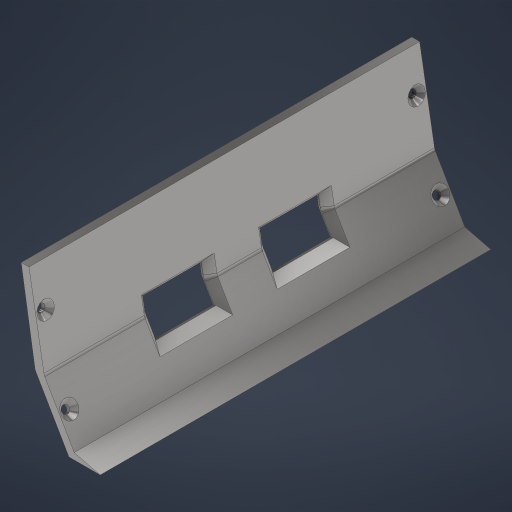
# Autodesk Inventor part: lemiesz
Saved by Autodesk Inventor 2024 (Build 280153000, 153)
## iProperties
Created: 2024-05-24
Part Number: lemiesz
Material: Steel
Document SubType Name: Modeling
Designer: Adam
Density: 7.85 g/cm^3
Appearance: Plate
Mass: 65.3515 g
Surface Area: 95.4294 cm^2
Volume: 8.32503 cm^3
Author: Adam
Autodesk Inventor part; units mm, degrees
ref_plane "YZ Plane" through (0, 0, 0) normal (1, 0, 0) x (0, 1, 0)
ref_plane "XZ Plane" through (0, 0, 0) normal (0, 1, 0) x (-1, 0, 0)
ref_plane "XY Plane" through (0, 0, 0) normal (0, 0, 1) x (1, 0, 0)
sketch "Sketch1" plane through (0, 0, 0) normal (0, 0, 1) x (1, 0, 0)
  line L0 (0, 0) -> (-8, 0)
  line L1 (-8, 0) -> (-16.4769, 14.6824)
  line L2 (0, 0) -> (-6.6505, 1.6626)
  line L3 (-14.1745, 14.6946) -> (-6.6505, 1.6626)
  line L4 (-14.4121, 15.3473) -> (-18.23, 37)
  line L5 (-14.3509, 15) -> (7.6359, 15) construction
  line L6 (-18.23, 37) -> (-20.23, 37)
  line L7 (-20.23, 37) -> (-16.719, 15.362)
  arc A0 (-16.719, 15.362) -> (-16.4769, 14.6824) centre (-14.7448, 15.6824) ccw
  arc A1 (-14.4121, 15.3473) -> (-14.1745, 14.6946) centre (-12.4425, 15.6946) ccw
  dimension "d0" = 8
  dimension "d1" = 120
  dimension "d3" = 2
  dimension "d37" = 100
  dimension "d38" = 2
  dimension "d39" = 2
  constraints: 16 end point, 4 point on circle, 4 tangent, 3 horizontal, 2 centre point, 2 point on line, 1 coincident, 1 equal length, 1 equal radius, 1 parallel
  measures "d0" distance of L0.start L1.start
  measures "d1" angle of L0 L1
  measures "d3" distance between parallel lines of L3 L1
  measures "d37" angle of L5 L4
  measures "d38" distance of L4.end L6.end
  measures "d39" radius of A0
extrude "Extrusion1" add sketch "Sketch1" along normal mid plane 100
sketch "Sketch6" plane through (0, 0, 0) normal (1, 0, 0) x (0, 1, 0)
  line L0 (1.6626, -50) -> (1.6626, 50) projected
  line L1 (17.6987, 22.5) -> (9.6987, 22.5)
  line L2 (9.6987, 22.5) -> (9.6987, 7.5)
  line L3 (9.6987, 7.5) -> (17.6987, 7.5)
  line L4 (17.6987, 7.5) -> (17.6987, 22.5)
  line L5 (17.6987, 22.5) -> (9.6987, 7.5) construction
  line L6 (9.6987, 22.5) -> (17.6987, 7.5) construction
  line L7 (17.6987, -7.5) -> (9.6987, -7.5)
  line L8 (9.6987, -7.5) -> (9.6987, -22.5)
  line L9 (9.6987, -22.5) -> (17.6987, -22.5)
  line L10 (17.6987, -22.5) -> (17.6987, -7.5)
  line L11 (17.6987, -7.5) -> (9.6987, -22.5) construction
  line L12 (9.6987, -7.5) -> (17.6987, -22.5) construction
  line L13 (1.6626, 50) -> (14.6946, 50) projected
  line L14 (14.6946, -50) -> (1.6626, -50) projected
  point P0 (0, 0)
  point P1 (37, 50)
  point P2 (34, 50)
  point P3 (13.6987, 15)
  point P4 (13.6987, -15)
  dimension "d22" = 8
  dimension "d23" = 15
  dimension "d24" = 8
  dimension "d25" = 15
  dimension "d40" = 35
  dimension "d41" = 35
  constraints: 24 end point, 4 midpoint, 4 parallel, 2 horizontal, 2 perpendicular
  measures "d22" distance of L3.end L2.end
  measures "d23" distance of L2.end L1.end
  measures "d24" distance of L9.end L8.end
  measures "d25" distance of L8.end L7.end
  measures "d40" distance from line of point (13.699, 15) L13
  measures "d41" distance from line of L14 point (13.699, -15)
extrude "Extrusion2" cut sketch "Sketch6" against normal through all
chamfer "Chamfer3" distance 1.8 angle 45 16 edges at (-12.7323, 12.1967, 22.5) (-14.3219, 15.0106, 22.5) (-14.6194, 16.523, 22.5) (-14.8267, 17.6987, 15) (-12.7323, 12.1967, 7.5) (-14.3219, 15.0106, 7.5) (-14.6194, 16.523, 7.5) (-11.2902, 9.6987, 15) (-12.7323, 12.1967, -7.5) (-14.3219, 15.0106, -7.5) (-14.6194, 16.523, -7.5) (-14.8267, 17.6987, -15) (-12.7323, 12.1967, -22.5) (-14.3219, 15.0106, -22.5) (-14.6194, 16.523, -22.5) (-11.2902, 9.6987, -15)
sketch "Sketch7" plane through (-18.23, 37, 50) normal (0.9848078, 0.1736482, 0) x (0, 0, -1)
  point P0 (50, -39.6035)
  point P1 (2.5, -10)
  point P2 (97.5, -10)
sketch "Sketch8" plane through (-6.6505, 1.6626, 50) normal (0.8660254, 0.5, 0) x (0, 0, -1)
  point P0 (50, -4.7651)
  point P1 (2.5, 7.5)
  point P2 (97.5, 7.5)
hole "Hole2" at (-16.4936, 27.1519, 47.5) at (-16.4936, 27.1519, -47.5) direction (-0.9848078, -0.1736482, 0) diameter 2 end through all
hole "Hole3" at (-10.4005, 8.1578, 47.5) at (-10.4005, 8.1578, -47.5) direction (-0.8660254, -0.5, 0) diameter 2 end through all
chamfer "Chamfer4" distance 1.2 angle 45 4 edges at (-16.4936, 27.1519, 48.5) (-10.4005, 8.1578, 46.5) (-16.4936, 27.1519, -46.5) (-10.4005, 8.1578, -48.5)
body "Solid1"
